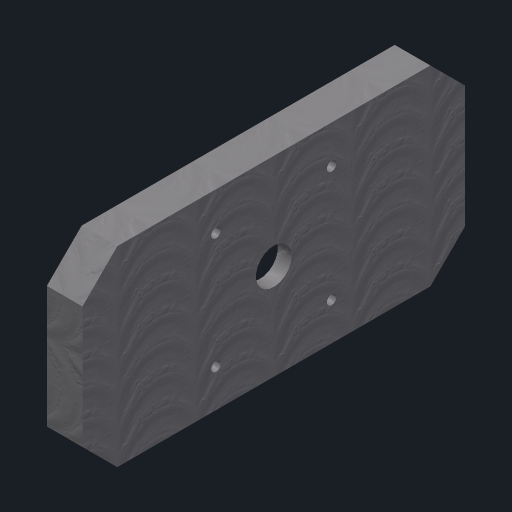
# Autodesk Inventor part: CAJA
Saved by Autodesk Inventor 2024.3 (Build 283343000, 343)
## iProperties
Created: 2024-06-29
Part Number: CAJA
Material: Steel, Mild, Welded
Document SubType Name: Modeling
Designer: Niler
Density: 7.85 g/cm^3
Appearance: Weld - Steel Mild
Author: Niler
Autodesk Inventor part; units mm, degrees
ref_plane "YZ Plane" through (0, 0, 0) normal (1, 0, 0) x (0, 1, 0)
ref_plane "XZ Plane" through (0, 0, 0) normal (0, 1, 0) x (-1, 0, 0)
ref_plane "XY Plane" through (0, 0, 0) normal (0, 0, 1) x (1, 0, 0)
sketch "Sketch1" plane through (0, 0, 0) normal (1, 0, 0) x (0, 1, 0)
  line L0 (-55, 110) -> (55, 110)
  line L1 (55, 110) -> (55, -110)
  line L2 (55, -110) -> (-55, -110)
  line L3 (-55, -110) -> (-55, 110)
  line L4 (-55, 110) -> (55, -110) construction
  line L5 (55, 110) -> (-55, -110) construction
  circle A0 centre (0, 57.5) radius 5
  circle A1 centre (0, -57.5) radius 5
  circle A2 centre (0, 0) radius 5
  line L6 (0, 57.5) -> (0, -57.5) construction
  line L7 (48, -103) -> (48, 103)
  line L8 (48, 103) -> (-48, 103)
  line L9 (-48, 103) -> (-48, -103)
  line L10 (-48, -103) -> (48, -103)
  dimension "d0" = 115
  dimension "d1" = 10
  dimension "d2" = 220
  dimension "d3" = 110
  dimension "d4" = 7
  constraints: 22 end point, 4 parallel, 3 centre point, 3 midpoint, 2 equal radius, 2 perpendicular, 2 vertical alignment, 1 coincident, 1 horizontal, 1 vertical, 3 other
  measures "d0" distance of L6.end L6.start
  measures "d1" diameter of A0
  measures "d2" distance between parallel lines of L2 L0
  measures "d3" distance of L0.start L0.end
  measures "d4" distance between parallel lines of L1 L7
extrude "Extrusion1" add sketch "Sketch1" along normal blind 8 contours L0 L1 L2 L3 | A0 | A1 | L10 L9 L8 L7
extrude "Extrusion2" add sketch "Sketch1" against normal blind 12.5 contours L0 L1 L2 L3 | A0 | A1
sketch "Sketch2" plane through (8, 0, 0) normal (1, 0, 0) x (0, 0, -1)
  line L0 (110, -55) -> (110, 55) projected
  line L1 (110, 55) -> (-110, 55) projected
  line L2 (-110, 55) -> (-110, -55) projected
  line L3 (-110, -55) -> (110, -55) projected
  circle A0 centre (0, 0) radius 5 projected
  line L4 (-33.234, -33.234) -> (33.234, -33.234) construction
  line L5 (33.234, -33.234) -> (33.234, 33.234) construction
  line L6 (33.234, 33.234) -> (-33.234, 33.234) construction
  line L7 (-33.234, 33.234) -> (-33.234, -33.234) construction
  line L8 (-33.234, -33.234) -> (33.234, 33.234) construction
  line L9 (33.234, -33.234) -> (-33.234, 33.234) construction
  circle A1 centre (0, 0) radius 47 construction
  circle A2 centre (33.234, 33.234) radius 2.75
  circle A3 centre (-33.234, 33.234) radius 2.75
  circle A4 centre (0, 0) radius 47 construction
  circle A5 centre (-33.234, -33.234) radius 2.75
  circle A6 centre (0, 0) radius 47 construction
  circle A7 centre (33.234, -33.234) radius 2.75
  circle A8 centre (0, 0) radius 47 construction
  dimension "d12" = 94
  dimension "d13" = 5.5
  dimension "d16" = 360
  constraints: 12 end point, 7 coincident, 4 centre point, 2 midpoint, 2 parallel, 2 perpendicular, 1 horizontal, 31 other
  measures "d13" diameter of A2
extrude "Extrusion3" cut sketch "Sketch2" against normal through all contours A2 | A3 | A5 | A7
sketch "Sketch3" plane through (0, 0, 0) normal (-1, 0, 0) x (0, 0, 1)
  circle A0 centre (33.234, -33.234) radius 2.75 projected
  circle A1 centre (33.234, 33.234) radius 2.75 projected
  circle A2 centre (-33.234, -33.234) radius 2.75 projected
  circle A3 centre (-33.234, 33.234) radius 2.75 projected
  line L0 (-103, -48) -> (103, -48) projected
  line L1 (103, -48) -> (103, 48) projected
  line L2 (103, 48) -> (-103, 48) projected
  line L3 (-103, 48) -> (-103, -48) projected
  circle A4 centre (57.5, 0) radius 5 projected
  circle A5 centre (-57.5, 0) radius 5 projected
  circle A6 centre (0, 0) radius 5 projected
  circle A7 centre (-33.234, 33.234) radius 4.5
  circle A8 centre (33.234, 33.234) radius 2.75 projected
  circle A9 centre (33.234, 33.234) radius 4.5
  circle A10 centre (-33.234, -33.234) radius 4.5
  circle A11 centre (33.234, -33.234) radius 4.5
  dimension "d20" = 9
  constraints: 4 centre point, 4 coincident, 3 equal radius
  measures "d20" diameter of A7
extrude "Extrusion4" cut sketch "Sketch3" against normal blind 3 contours A0 | A1 | A2 | A3 | A7 | A9 | A10 | A11
fillet "Fillet1" radius 2 2 edges at (0, -5, -57.5) (0, -5, 57.5)
sketch "Sketch4" plane through (8, 0, 0) normal (1, 0, 0) x (0, 0, -1)
  circle A0 centre (-33.234, -33.234) radius 2.75 projected
  circle A1 centre (-33.234, 33.234) radius 2.75 projected
  circle A2 centre (33.234, -33.234) radius 2.75 projected
  circle A3 centre (33.234, 33.234) radius 2.75 projected
  line L0 (110, -55) -> (110, 55) projected
  line L1 (110, 55) -> (-110, 55) projected
  line L2 (-110, 55) -> (-110, -55) projected
  line L3 (-110, -55) -> (110, -55) projected
  circle A4 centre (0, 0) radius 5 projected
  circle A5 centre (0, 0) radius 10.3
  dimension "d24" = 20.6
  constraints: 1 centre point, 1 coincident
  measures "d24" diameter of A5
extrude "Extrusion5" cut sketch "Sketch4" against normal through all contours A4 | A5
sketch "Sketch5" plane through (-12.5, 0, -57.5) normal (-1, 0, 0) x (0, 0, 1)
  circle A0 centre (0, 0) radius 5 projected
  circle A1 centre (115, 0) radius 5 projected
  point P0 (57.5, 0)
extrude "Extrusion6" cut sketch "Sketch5" against normal blind 2.5
chamfer "Chamfer2" distance 20 angle 45 8 edges at (-6.25, 48, -103) (-6.25, -48, -103) (-6.25, -48, 103) (-6.25, 48, 103) (-2.25, 55, -110) (-2.25, -55, -110) (-2.25, -55, 110) (-2.25, 55, 110)
body "Solid1"
